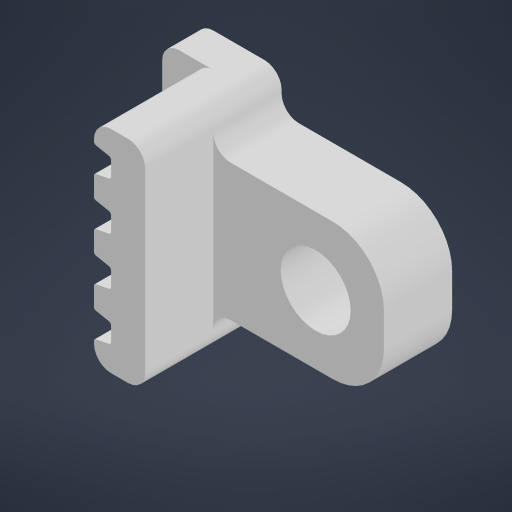
# Autodesk Inventor part: PoleClip
Saved by Autodesk Inventor 2023 (Build 270158000, 158)
## iProperties
Created: 2023-03-14
Part Number: PoleClip
Material: Generic
Document SubType Name: Modeling
Designer: Matt
Density: 1 g/cm^3
Appearance: Default
Author: Matt
Autodesk Inventor part; units mm, degrees
ref_plane "YZ Plane" through (0, 0, 0) normal (1, 0, 0) x (0, 1, 0)
ref_plane "XZ Plane" through (0, 0, 0) normal (0, 1, 0) x (-1, 0, 0)
ref_plane "XY Plane" through (0, 0, 0) normal (0, 0, 1) x (1, 0, 0)
sketch "Sketch2" plane through (0, 0, 0) normal (0, 0, 1) x (1, 0, 0)
  line L0 (2, 16.6) -> (2, 17.7)
  arc A0 (2.0995, 17.8199) -> (2, 17.7) centre (2.1238, 17.6985) ccw
  line L1 (2.0995, 17.8199) -> (2.899, 17.9798)
  arc A1 (2.899, 17.9798) -> (3, 18.1306) centre (2.837, 18.1306) ccw
  line L2 (3, 18.1306) -> (3, 18.9694)
  arc A2 (3, 18.9694) -> (2.899, 19.1202) centre (2.837, 18.9694) ccw
  line L3 (2.899, 19.1202) -> (2.0995, 19.2801)
  arc A3 (2, 19.4) -> (2.0995, 19.2801) centre (2.1238, 19.4015) ccw
  line L4 (2, 19.4) -> (2, 20.5)
  arc A4 (2.0995, 20.6199) -> (2, 20.5) centre (2.1238, 20.4985) ccw
  line L5 (2.0995, 20.6199) -> (2.899, 20.7798)
  arc A5 (2.899, 20.7798) -> (3, 20.9306) centre (2.837, 20.9306) ccw
  line L6 (3, 20.9306) -> (3, 21.7694)
  arc A6 (3, 21.7694) -> (2.899, 21.9202) centre (2.837, 21.7694) ccw
  line L7 (2.899, 21.9202) -> (2.0995, 22.0801)
  arc A7 (2, 22.2) -> (2.0995, 22.0801) centre (2.1238, 22.2015) ccw
  line L8 (2, 22.2) -> (2, 23.3)
  arc A8 (2.0995, 23.4199) -> (2, 23.3) centre (2.1238, 23.2985) ccw
  line L9 (2.0995, 23.4199) -> (2.899, 23.5798)
  arc A9 (2.899, 23.5798) -> (3, 23.7306) centre (2.837, 23.7306) ccw
  line L10 (3, 23.7306) -> (3, 24.5694)
  arc A10 (3, 24.5694) -> (2.899, 24.7202) centre (2.837, 24.5694) ccw
  line L11 (2.899, 24.7202) -> (2.0995, 24.8801)
  arc A11 (2, 25) -> (2.0995, 24.8801) centre (2.1238, 25.0015) ccw
  line L12 (2, 25) -> (2, 26.1)
  arc A12 (2.0995, 26.2199) -> (2, 26.1) centre (2.1238, 26.0985) ccw
  line L13 (2.0995, 26.2199) -> (2.899, 26.3798)
  arc A13 (2.899, 26.3798) -> (3, 26.5306) centre (2.837, 26.5306) ccw
  line L14 (3, 26.5306) -> (3, 27.3694)
  arc A14 (3, 27.3694) -> (2.899, 27.5202) centre (2.837, 27.3694) ccw
  line L15 (2.899, 27.5202) -> (2.0995, 27.6801)
  arc A15 (2, 27.8) -> (2.0995, 27.6801) centre (2.1238, 27.8015) ccw
  line L16 (2, 27.8) -> (2, 28.9)
  arc A16 (2.0995, 29.0199) -> (2, 28.9) centre (2.1238, 28.8985) ccw
  line L17 (2.0995, 29.0199) -> (2.899, 29.1798)
  arc A17 (2.899, 29.1798) -> (3, 29.3306) centre (2.837, 29.3306) ccw
  line L18 (3, 29.3306) -> (3, 30.1694)
  arc A18 (3, 30.1694) -> (2.899, 30.3202) centre (2.837, 30.1694) ccw
  line L19 (2.899, 30.3202) -> (2.0995, 30.4801)
  arc A19 (2, 30.6) -> (2.0995, 30.4801) centre (2.1238, 30.6015) ccw
  line L20 (2, 30.6) -> (2, 31.7)
  arc A20 (2.0995, 31.8199) -> (2, 31.7) centre (2.1238, 31.6985) ccw
  line L21 (2.0995, 31.8199) -> (2.899, 31.9798)
  arc A21 (2.899, 31.9798) -> (3, 32.1306) centre (2.837, 32.1306) ccw
  line L22 (3, 32.1306) -> (3, 32.9694)
  arc A22 (3, 32.9694) -> (2.899, 33.1202) centre (2.837, 32.9694) ccw
  line L23 (2.899, 33.1202) -> (2.0995, 33.2801)
  arc A23 (2, 33.4) -> (2.0995, 33.2801) centre (2.1238, 33.4015) ccw
  line L24 (2, 33.4) -> (2, 34.5)
  arc A24 (2.0995, 34.6199) -> (2, 34.5) centre (2.1238, 34.4985) ccw
  line L25 (2.0995, 34.6199) -> (2.899, 34.7798)
  arc A25 (2.899, 34.7798) -> (3, 34.9306) centre (2.837, 34.9306) ccw
  line L26 (3, 34.9306) -> (3, 35.7694)
  arc A26 (3, 35.7694) -> (2.899, 35.9202) centre (2.837, 35.7694) ccw
  line L27 (2.899, 35.9202) -> (2.0995, 36.0801)
  arc A27 (2, 36.2) -> (2.0995, 36.0801) centre (2.1238, 36.2015) ccw
  line L28 (2, 36.2) -> (2, 37.3)
  arc A28 (2.0995, 37.4199) -> (2, 37.3) centre (2.1238, 37.2985) ccw
  line L29 (2.0995, 37.4199) -> (2.899, 37.5798)
  arc A29 (2.899, 37.5798) -> (3, 37.7306) centre (2.837, 37.7306) ccw
  line L30 (3, 37.7306) -> (3, 38.5694)
  arc A30 (3, 38.5694) -> (2.899, 38.7202) centre (2.837, 38.5694) ccw
  line L31 (2.899, 38.7202) -> (2.0995, 38.8801)
  arc A31 (2, 39) -> (2.0995, 38.8801) centre (2.1238, 39.0015) ccw
  line L32 (2, 39) -> (2, 40.1)
  arc A32 (2.0995, 40.2199) -> (2, 40.1) centre (2.1238, 40.0985) ccw
  line L33 (2.0995, 40.2199) -> (2.899, 40.3798)
  arc A33 (2.899, 40.3798) -> (3, 40.5306) centre (2.837, 40.5306) ccw
  line L34 (3, 40.5306) -> (3, 41.3694)
  arc A34 (3, 41.3694) -> (2.899, 41.5202) centre (2.837, 41.3694) ccw
  line L35 (2.899, 41.5202) -> (2.0995, 41.6801)
  arc A35 (2, 41.8) -> (2.0995, 41.6801) centre (2.1238, 41.8015) ccw
  line L36 (2, 41.8) -> (2, 42.9)
  arc A36 (2.0995, 43.0199) -> (2, 42.9) centre (2.1238, 42.8985) ccw
  line L37 (2.0995, 43.0199) -> (2.899, 43.1798)
  arc A37 (2.899, 43.1798) -> (3, 43.3306) centre (2.837, 43.3306) ccw
  line L38 (3, 43.3306) -> (3, 44.1694)
  arc A38 (3, 44.1694) -> (2.899, 44.3202) centre (2.837, 44.1694) ccw
  line L39 (2.899, 44.3202) -> (2.0995, 44.4801)
  arc A39 (2, 44.6) -> (2.0995, 44.4801) centre (2.1238, 44.6015) ccw
  line L40 (2, 44.6) -> (2, 45.7)
  arc A40 (2.0995, 45.8199) -> (2, 45.7) centre (2.1238, 45.6985) ccw
  line L41 (2.0995, 45.8199) -> (2.899, 45.9798)
  arc A41 (2.899, 45.9798) -> (3, 46.1306) centre (2.837, 46.1306) ccw
  line L42 (3, 46.1306) -> (3, 46.9694)
  arc A42 (3, 46.9694) -> (2.899, 47.1202) centre (2.837, 46.9694) ccw
  line L43 (2.899, 47.1202) -> (2.0995, 47.2801)
  arc A43 (2, 47.4) -> (2.0995, 47.2801) centre (2.1238, 47.4015) ccw
  line L44 (2, 47.4) -> (2, 48.5)
  arc A44 (2.0995, 48.6199) -> (2, 48.5) centre (2.1238, 48.4985) ccw
  line L45 (2.0995, 48.6199) -> (2.899, 48.7798)
  arc A45 (2.899, 48.7798) -> (3, 48.9306) centre (2.837, 48.9306) ccw
  line L46 (3, 48.9306) -> (3, 49.7694)
  arc A46 (3, 49.7694) -> (2.899, 49.9202) centre (2.837, 49.7694) ccw
  line L47 (2.899, 49.9202) -> (2.0995, 50.0801)
  arc A47 (2, 50.2) -> (2.0995, 50.0801) centre (2.1238, 50.2015) ccw
  line L48 (2, 50.2) -> (2, 51.3)
  arc A48 (2.0995, 51.4199) -> (2, 51.3) centre (2.1238, 51.2985) ccw
  line L49 (2.0995, 51.4199) -> (2.899, 51.5798)
  arc A49 (2.899, 51.5798) -> (3, 51.7306) centre (2.837, 51.7306) ccw
  line L50 (3, 51.7306) -> (3, 52.5694)
  arc A50 (3, 52.5694) -> (2.899, 52.7202) centre (2.837, 52.5694) ccw
  line L51 (2.899, 52.7202) -> (2.0995, 52.8801)
  arc A51 (2, 53) -> (2.0995, 52.8801) centre (2.1238, 53.0015) ccw
  line L52 (2, 53) -> (2, 54.1)
  arc A52 (2.0995, 54.2199) -> (2, 54.1) centre (2.1238, 54.0985) ccw
  line L53 (2.0995, 54.2199) -> (2.899, 54.3798)
  arc A53 (2.899, 54.3798) -> (3, 54.5306) centre (2.837, 54.5306) ccw
  line L54 (3, 54.5306) -> (3, 55.3694)
  arc A54 (3, 55.3694) -> (2.899, 55.5202) centre (2.837, 55.3694) ccw
  line L55 (2.899, 55.5202) -> (2.0995, 55.6801)
  arc A55 (2, 55.8) -> (2.0995, 55.6801) centre (2.1238, 55.8015) ccw
  line L56 (2, 55.8) -> (2, 56.9)
  arc A56 (2.0995, 57.0199) -> (2, 56.9) centre (2.1238, 56.8985) ccw
  line L57 (2.0995, 57.0199) -> (2.899, 57.1798)
  arc A57 (2.899, 57.1798) -> (3, 57.3306) centre (2.837, 57.3306) ccw
  line L58 (3, 57.3306) -> (3, 58.1694)
  arc A58 (3, 58.1694) -> (2.899, 58.3202) centre (2.837, 58.1694) ccw
  line L59 (2.899, 58.3202) -> (2.0995, 58.4801)
  arc A59 (2, 58.6) -> (2.0995, 58.4801) centre (2.1238, 58.6015) ccw
  line L60 (2, 58.6) -> (2, 59.7)
  arc A60 (2.0995, 59.8199) -> (2, 59.7) centre (2.1238, 59.6985) ccw
  line L61 (2.0995, 59.8199) -> (2.899, 59.9798)
  arc A61 (2.899, 59.9798) -> (3, 60.1306) centre (2.837, 60.1306) ccw
  line L62 (3, 60.1306) -> (3, 60.9694)
  arc A62 (3, 60.9694) -> (2.899, 61.1202) centre (2.837, 60.9694) ccw
  line L63 (2.899, 61.1202) -> (2.0995, 61.2801)
  arc A63 (2, 61.4) -> (2.0995, 61.2801) centre (2.1238, 61.4015) ccw
  line L64 (2, 61.4) -> (2, 62.5)
  arc A64 (2.0995, 62.6199) -> (2, 62.5) centre (2.1238, 62.4985) ccw
  line L65 (2.0995, 62.6199) -> (2.899, 62.7798)
  arc A65 (2.899, 62.7798) -> (3, 62.9306) centre (2.837, 62.9306) ccw
  line L66 (3, 62.9306) -> (3, 63.7694)
  arc A66 (3, 63.7694) -> (2.899, 63.9202) centre (2.837, 63.7694) ccw
  line L67 (2.899, 63.9202) -> (2.0995, 64.0801)
  arc A67 (2, 64.2) -> (2.0995, 64.0801) centre (2.1238, 64.2015) ccw
  line L68 (2, 64.2) -> (2, 65.3)
  arc A68 (2.0995, 65.4199) -> (2, 65.3) centre (2.1238, 65.2985) ccw
  line L69 (2.0995, 65.4199) -> (2.899, 65.5798)
  arc A69 (2.899, 65.5798) -> (3, 65.7306) centre (2.837, 65.7306) ccw
  line L70 (3, 65.7306) -> (3, 66.5694)
  arc A70 (3, 66.5694) -> (2.899, 66.7202) centre (2.837, 66.5694) ccw
  line L71 (2.899, 66.7202) -> (2.0995, 66.8801)
  arc A71 (2, 67) -> (2.0995, 66.8801) centre (2.1238, 67.0015) ccw
  line L72 (2, 67) -> (2, 68.1)
  arc A72 (2.0995, 68.2199) -> (2, 68.1) centre (2.1238, 68.0985) ccw
  line L73 (2.0995, 68.2199) -> (2.899, 68.3798)
  arc A73 (2.899, 68.3798) -> (3, 68.5306) centre (2.837, 68.5306) ccw
  line L74 (3, 68.5306) -> (3, 69.3694)
  arc A74 (3, 69.3694) -> (2.899, 69.5202) centre (2.837, 69.3694) ccw
  line L75 (2.899, 69.5202) -> (2.0995, 69.6801)
  arc A75 (2, 69.8) -> (2.0995, 69.6801) centre (2.1238, 69.8015) ccw
  line L76 (2, 69.8) -> (2, 70.9)
  arc A76 (2.0995, 71.0199) -> (2, 70.9) centre (2.1238, 70.8985) ccw
  line L77 (2.0995, 71.0199) -> (2.899, 71.1798)
  arc A77 (2.899, 71.1798) -> (3, 71.3306) centre (2.837, 71.3306) ccw
  line L78 (3, 71.3306) -> (3, 72.1694)
  arc A78 (3, 72.1694) -> (2.899, 72.3202) centre (2.837, 72.1694) ccw
  line L79 (2.899, 72.3202) -> (2.0995, 72.4801)
  arc A79 (2, 72.6) -> (2.0995, 72.4801) centre (2.1238, 72.6015) ccw
  line L80 (2, 72.6) -> (2, 73.7)
  arc A80 (2.0995, 73.8199) -> (2, 73.7) centre (2.1238, 73.6985) ccw
  line L81 (2.0995, 73.8199) -> (2.899, 73.9798)
  arc A81 (2.899, 73.9798) -> (3, 74.1306) centre (2.837, 74.1306) ccw
  line L82 (3, 74.1306) -> (3, 74.9694)
  arc A82 (3, 74.9694) -> (2.899, 75.1202) centre (2.837, 74.9694) ccw
  line L83 (2.899, 75.1202) -> (2.0995, 75.2801)
  arc A83 (2, 75.4) -> (2.0995, 75.2801) centre (2.1238, 75.4015) ccw
  line L84 (2, 75.4) -> (2, 76.5)
  arc A84 (2.0995, 76.6199) -> (2, 76.5) centre (2.1238, 76.4985) ccw
  line L85 (2.0995, 76.6199) -> (2.899, 76.7798)
  arc A85 (2.899, 76.7798) -> (3, 76.9306) centre (2.837, 76.9306) ccw
  line L86 (3, 76.9306) -> (3, 77.7694)
  arc A86 (3, 77.7694) -> (2.899, 77.9202) centre (2.837, 77.7694) ccw
  line L87 (2.899, 77.9202) -> (2.0995, 78.0801)
  arc A87 (2, 78.2) -> (2.0995, 78.0801) centre (2.1238, 78.2015) ccw
  line L88 (2, 78.2) -> (2, 79.3)
  arc A88 (2.0995, 79.4199) -> (2, 79.3) centre (2.1238, 79.2985) ccw
  line L89 (2.0995, 79.4199) -> (2.899, 79.5798)
  arc A89 (2.899, 79.5798) -> (3, 79.7306) centre (2.837, 79.7306) ccw
  line L90 (3, 79.7306) -> (3, 80.5694)
  arc A90 (3, 80.5694) -> (2.899, 80.7202) centre (2.837, 80.5694) ccw
  line L91 (2.899, 80.7202) -> (2.0995, 80.8801)
  arc A91 (2, 81) -> (2.0995, 80.8801) centre (2.1238, 81.0015) ccw
  line L92 (2, 81) -> (2, 82.1)
  arc A92 (2.0995, 82.2199) -> (2, 82.1) centre (2.1238, 82.0985) ccw
  line L93 (2.0995, 82.2199) -> (2.899, 82.3798)
  arc A93 (2.899, 82.3798) -> (3, 82.5306) centre (2.837, 82.5306) ccw
  line L94 (3, 82.5306) -> (3, 83.3694)
  arc A94 (3, 83.3694) -> (2.899, 83.5202) centre (2.837, 83.3694) ccw
  line L95 (2.899, 83.5202) -> (2.0995, 83.6801)
  arc A95 (2, 83.8) -> (2.0995, 83.6801) centre (2.1238, 83.8015) ccw
  line L96 (2, 83.8) -> (2, 84.9)
  arc A96 (2.0995, 85.0199) -> (2, 84.9) centre (2.1238, 84.8985) ccw
  line L97 (2.0995, 85.0199) -> (2.899, 85.1798)
  arc A97 (2.899, 85.1798) -> (3, 85.3306) centre (2.837, 85.3306) ccw
  line L98 (3, 85.3306) -> (3, 86.1694)
  arc A98 (3, 86.1694) -> (2.899, 86.3202) centre (2.837, 86.1694) ccw
  line L99 (2.899, 86.3202) -> (2.0995, 86.4801)
  arc A99 (2, 86.6) -> (2.0995, 86.4801) centre (2.1238, 86.6015) ccw
  line L100 (2, 86.6) -> (2, 87.7)
  arc A100 (2.0995, 87.8199) -> (2, 87.7) centre (2.1238, 87.6985) ccw
  line L101 (2.0995, 87.8199) -> (2.899, 87.9798)
  arc A101 (2.899, 87.9798) -> (3, 88.1306) centre (2.837, 88.1306) ccw
  line L102 (3, 88.1306) -> (3, 88.9694)
  arc A102 (3, 88.9694) -> (2.899, 89.1202) centre (2.837, 88.9694) ccw
  line L103 (2.899, 89.1202) -> (2.0995, 89.2801)
  arc A103 (2, 89.4) -> (2.0995, 89.2801) centre (2.1238, 89.4015) ccw
  line L104 (2, 89.4) -> (2, 90.5)
  arc A104 (2.0995, 90.6199) -> (2, 90.5) centre (2.1238, 90.4985) ccw
  line L105 (2.0995, 90.6199) -> (2.899, 90.7798)
  arc A105 (2.899, 90.7798) -> (3, 90.9306) centre (2.837, 90.9306) ccw
  line L106 (3, 90.9306) -> (3, 91.7694)
  arc A106 (3, 91.7694) -> (2.899, 91.9202) centre (2.837, 91.7694) ccw
  line L107 (2.899, 91.9202) -> (2.0995, 92.0801)
  arc A107 (2, 92.2) -> (2.0995, 92.0801) centre (2.1238, 92.2015) ccw
  line L108 (2, 92.2) -> (2, 93.3)
  arc A108 (2.0995, 93.4199) -> (2, 93.3) centre (2.1238, 93.2985) ccw
  line L109 (2.0995, 93.4199) -> (2.899, 93.5798)
  arc A109 (2.899, 93.5798) -> (3, 93.7306) centre (2.837, 93.7306) ccw
  line L110 (3, 93.7306) -> (3, 94.5694)
  arc A110 (3, 94.5694) -> (2.899, 94.7202) centre (2.837, 94.5694) ccw
  line L111 (2.899, 94.7202) -> (2.0995, 94.8801)
  arc A111 (2, 95) -> (2.0995, 94.8801) centre (2.1238, 95.0015) ccw
  line L112 (2, 95) -> (2, 96.1)
  arc A112 (2.0995, 96.2199) -> (2, 96.1) centre (2.1238, 96.0985) ccw
  line L113 (2.0995, 96.2199) -> (2.899, 96.3798)
  arc A113 (2.899, 96.3798) -> (3, 96.5306) centre (2.837, 96.5306) ccw
  line L114 (3, 96.5306) -> (3, 97.3694)
  arc A114 (3, 97.3694) -> (2.899, 97.5202) centre (2.837, 97.3694) ccw
  line L115 (2.899, 97.5202) -> (2.0995, 97.6801)
  arc A115 (2, 97.8) -> (2.0995, 97.6801) centre (2.1238, 97.8015) ccw
  line L116 (2, 97.8) -> (2, 99.5)
  arc A116 (2, 99.5) -> (1.5, 100) centre (1.5, 99.5) ccw
  line L117 (1.5, 100) -> (0.5, 100)
  arc A117 (0.5, 100) -> (0, 99.5) centre (0.5, 99.5) ccw
  line L118 (0, 99.5) -> (0, 1)
  arc A118 (0, 1) -> (1, 0) centre (1, 1) ccw
  line L119 (1, 0) -> (7, 0)
  arc A119 (7, 0) -> (8, 1) centre (7, 1) ccw
  line L120 (8, 1) -> (8, 9)
  arc A120 (8, 9) -> (7, 10) centre (7, 9) ccw
  arc A121 (2.0008, 14.9123) -> (7, 10) centre (7, 15) ccw
  arc A122 (2.0995, 15.0199) -> (2.0008, 14.9123) centre (2.1238, 14.8985) ccw
  line L121 (2.0995, 15.0199) -> (2.899, 15.1798)
  arc A123 (2.899, 15.1798) -> (3, 15.3306) centre (2.837, 15.3306) ccw
  line L122 (3, 15.3306) -> (3, 16.1694)
  arc A124 (3, 16.1694) -> (2.899, 16.3202) centre (2.837, 16.1694) ccw
  line L123 (2.899, 16.3202) -> (2.0995, 16.4801)
  arc A125 (2, 16.6) -> (2.0995, 16.4801) centre (2.1238, 16.6015) ccw
  circle A126 centre (3, 6) radius 1.55
  line L124 (2, 96.95) -> (14, 96.95)
  line L125 (14, 96.95) -> (14, 88.55)
  line L126 (14, 88.55) -> (2, 88.55)
  line L127 (2, 88.55) -> (2, 96.95)
  line L128 (2, 96.95) -> (5, 96.95)
  line L129 (5, 96.95) -> (5, 98.95)
  line L130 (5, 98.95) -> (2, 98.95)
  line L131 (2, 98.95) -> (2, 96.95)
  line L132 (2, 88.55) -> (5, 88.55)
  line L133 (5, 88.55) -> (5, 86.55)
  line L134 (5, 86.55) -> (2, 86.55)
  line L135 (2, 86.55) -> (2, 88.55)
  line L136 (5, 96.95) -> (5, 88.55)
  point P0 (0, 0)
  point P1 (0, 0)
  point P2 (3, 88.55)
  point P3 (3, 96.95)
  dimension "d9" = 12
  dimension "d12" = 3
  dimension "d13" = 2
  dimension "d14" = 3
  dimension "d15" = 2
  constraints: 274 end point, 252 point on circle, 127 centre point, 6 parallel, 3 horizontal, 3 perpendicular
  measures "d9" distance of L125.end L126.end
  measures "d12" distance of L130.end L129.end
  measures "d13" distance of L129.end L128.end
  measures "d14" distance of L133.end L134.end
  measures "d15" distance of L132.end L133.end
extrude "Extrusion2" add sketch "Sketch2" along normal blind 6 contours L130 L129 L124 L114 A114 L115 A115 L116 | L136 L126 L102 A102 L103 A103 L104 A104 L105 A105 L106 A106 L107 A107 L108 A108 L109 A109 L110 A110 L111 A111 L112 A112 L113 A113 L114 L124 | L133 L134 A99 L100 A100 L101 A101 L102 L126 | L134 L135 A99
sketch "Sketch4" plane through (0, 0, 0) normal (0, 0, -1) x (-1, 0, 0)
  line L0 (-5, 86.55) -> (-5, 98.95) projected
  line L1 (-5, 86.55) -> (0, 86.55)
  line L2 (0, 86.55) -> (0, 98.95)
  line L3 (0, 98.95) -> (-5, 98.95)
  line L4 (-5, 98.95) -> (-5, 86.55)
  point P0 (0, 0)
  constraints: 8 end point, 2 parallel, 1 horizontal, 1 perpendicular
extrude "Extrusion3" add sketch "Sketch4" along normal blind 2
sketch "Sketch5" plane through (0, 0, -2) normal (0, 0, -1) x (-1, 0, 0)
  line L0 (-5, 86.55) -> (-5, 98.95) projected
  line L1 (-5, 92.75) -> (-15, 92.75)
  line L2 (-15, 92.75) -> (-15, 88.75)
  line L3 (-15, 88.75) -> (-5, 88.75)
  line L4 (-5, 88.75) -> (-5, 92.75)
  line L5 (-5, 98.95) -> (-5, 86.55)
  line L6 (-15, 92.75) -> (-15, 96.75)
  line L7 (-15, 96.75) -> (-5, 96.75)
  line L8 (-5, 96.75) -> (-5, 92.75)
  circle A0 centre (-11, 92.75) radius 2.05
  point P0 (0, 0)
  dimension "d18" = 10
  dimension "d19" = 4
  dimension "d20" = 4.1
  dimension "d21" = 4
  constraints: 16 end point, 4 symmetric about line, 2 parallel, 1 centre point, 1 horizontal, 1 midpoint, 1 perpendicular, 1 point on line
  measures "d18" distance of L3.end L2.end
  measures "d19" distance of L2.end L1.end
  measures "d20" diameter of A0
  measures "d21" distance from line of L2 A0.centre
extrude "Extrusion4" add sketch "Sketch5" against normal blind 4 contours L3 L2 L1 A0 L0 | L1 A0 L6 L7 L0
fillet "Fillet1" radius 1 8 edges at (2, 98.95, 3) (0, 98.95, -1) (5, 98.95, 2) (5, 96.75, 0) (5, 86.55, 2) (5, 88.75, 0) (2, 86.55, 3) (0, 86.55, -1)
fillet "Fillet1" radius 3 2 edges at (15, 96.75, 0) (15, 88.75, 0)
body "Solid2"
